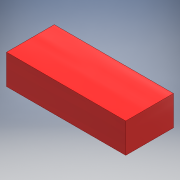
# Autodesk Inventor part: 回路
Saved by Autodesk Inventor 2017 (Build 210142000, 142)
## iProperties
Part Number: 回路
Material: 一般
Document SubType Name: Modeling
Designer: 雪村
Density: 0.75 g/cm^3
Appearance: 淡い赤
Mass: 75 g
Surface Area: 150 cm^2
Volume: 100 cm^3
Author: 雪村
Autodesk Inventor part; units mm, degrees
ref_plane "YZ Plane" through (0, 0, 0) normal (1, 0, 0) x (0, 1, 0)
ref_plane "XZ Plane" through (0, 0, 0) normal (0, 1, 0) x (-1, 0, 0)
ref_plane "XY Plane" through (0, 0, 0) normal (0, 0, 1) x (1, 0, 0)
sketch "スケッチ1" plane through (0, 0, 0) normal (0, 0, 1) x (1, 0, 0)
  line L0 (0, 0) -> (100, 0)
  line L1 (100, 0) -> (100, 40)
  line L2 (100, 40) -> (0, 40)
  line L3 (0, 40) -> (0, 0)
  dimension "d0" = 100
  dimension "d1" = 40
  constraints: 8 end point
  measures "d0" distance of L2.end L1.end
  measures "d1" distance of L1.end L0.end
extrude "押し出し1" add sketch "スケッチ1" along normal blind 25
